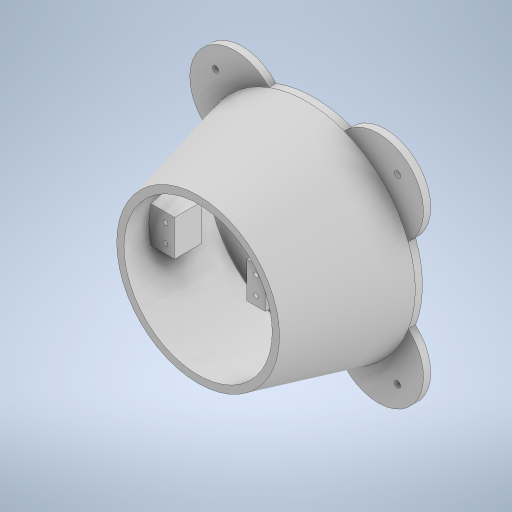
# Autodesk Inventor part: arm_base
Saved by Autodesk Inventor 2023 (Build 270158000, 158)
## iProperties
Created: 2023-01-17
Part Number: arm_base
Material: Generic
Document SubType Name: Modeling
Designer: denyh
Density: 1 g/cm^3
Appearance: Default
Author: denyh
Autodesk Inventor part; units mm, degrees
ref_plane "YZ Plane" through (0, 0, 0) normal (1, 0, 0) x (0, 1, 0)
ref_plane "XZ Plane" through (0, 0, 0) normal (0, 1, 0) x (-1, 0, 0)
ref_plane "Work Plane1" through (0, 0, 64) normal (0, 0, 1) x (1, 0, 0)
sketch "Sketch5" plane through (0, 0, 0) normal (0, 0, 1) x (1, 0, 0)
  circle A0 centre (0, 0) radius 60 projected
  line L0 (0, -6) -> (55.6072, -6) construction
  line L1 (0, 6) -> (55.6072, 6) construction
  arc A1 (-36.4842, -42.4842) -> (-36.4842, 42.4842) centre (0, 0) ccw
  circle A2 centre (0, 0) radius 56
  dimension "d15" = 6
  dimension "d16" = 12
  constraints: 4 end point, 2 horizontal, 2 point on circle, 1 centre point, 1 coincident, 3 other
  measures "d15" distance of A0.centre L1.start
  measures "d16" distance of L1.start L0.start
extrude "Extrusion1" add sketch "Sketch5" along normal blind 4 contours A0 | A2 A1
sketch "Sketch6" plane through (0, 0, 64) normal (0, 0, 1) x (1, 0, 0)
  circle A0 centre (0, 0) radius 45
  dimension "d22" = 90
  constraints: 1 centre point, 1 coincident
  measures "d22" diameter of A0
loft "Loft3" add profiles "Sketch6" section 1 edges at (-60, 0, 4)
sketch "Sketch9" plane through (0, 0, 64) normal (0, 0, 1) x (1, 0, 0)
  circle A0 centre (0, 0) radius 41
  dimension "d28" = 82
  constraints: 1 centre point, 1 coincident
  measures "d28" diameter of A0
sketch "Sketch10" plane through (0, 0, 0) normal (0, 0, -1) x (-1, 0, 0)
  circle A0 centre (0, 0) radius 56
  dimension "d29" = 112
  constraints: 1 centre point, 1 coincident
  measures "d29" diameter of A0
loft "Loft4" cut profiles "Sketch10", "Sketch9"
sketch "Sketch11" plane through (0, 0, 0) normal (0, 0, -1) x (-1, 0, 0)
  line L0 (0, 0) -> (0, 6)
  line L1 (0, 6) -> (-36.4842, 42.4842)
  circle A0 centre (0, 0) radius 56 projected
  line L2 (0, 0) -> (0, -6)
  line L3 (0, -6) -> (-36.4842, -42.4842)
  arc A1 (-36.4842, 42.4842) -> (-36.4842, -42.4842) centre (0, 0) ccw
  dimension "d34" = 6
  dimension "d35" = 135
  dimension "d36" = 6
  dimension "d37" = 135
  constraints: 8 end point, 4 point on circle, 2 vertical, 1 centre point, 1 coincident, 1 concentric
  measures "d34" distance of L0.start L0.end
  measures "d35" angle of L1 L0
  measures "d36" distance of L2.start L2.end
  measures "d37" angle of L2 L3
extrude "Extrusion2" add sketch "Sketch11" against normal blind 4 contours L2 L3 A0 L1 L0 picked at (-37.0571, 3.1994)
sketch "Sketch13" plane through (0, 0, 4) normal (0, 0, 1) x (1, 0, 0)
  line L0 (0, 0) -> (14, 0)
  line L1 (14, 0) -> (19, 0)
  line L2 (19, 0) -> (19, -10)
  line L3 (19, -10) -> (9, -10)
  line L4 (9, -10) -> (9, 10)
  line L5 (9, 10) -> (19, 10)
  line L6 (19, 10) -> (19, 0)
  dimension "d46" = 14
  dimension "d47" = 5
  dimension "d48" = 10
  dimension "d49" = 10
  dimension "d50" = 20
  constraints: 14 end point, 5 perpendicular, 2 point on line, 1 horizontal
  measures "d46" distance of L0.start L0.end
  measures "d47" distance of L0.end L1.end
  measures "d48" distance of L1.end L2.end
  measures "d49" distance of L2.end L3.end
  measures "d50" distance of L3.end L4.end
extrude "Extrusion3" add sketch "Sketch13" along normal blind 42
sketch "Sketch14" plane through (0, 0, 46) normal (0, 0, 1) x (1, 0, 0)
  line L0 (0, 0) -> (14, 0)
  line L1 (14, 0) -> (14, -5)
  circle A0 centre (14, -5) radius 1.3
  line L2 (14, 0) -> (14, 5)
  circle A1 centre (14, 5) radius 1.3
  dimension "d53" = 14
  dimension "d54" = 5
  dimension "d55" = 2.6
  dimension "d56" = 5
  dimension "d57" = 2.6
  constraints: 6 end point, 2 centre point, 2 coincident, 1 horizontal, 1 perpendicular, 1 vertical
  measures "d53" distance of L0.start L0.end
  measures "d54" distance of L0.end L1.end
  measures "d55" diameter of A0
  measures "d56" distance of L0.end L2.end
  measures "d57" diameter of A1
extrude "Extrusion4" cut sketch "Sketch14" against normal blind 10
sketch "Sketch15" plane through (0, 0, 4) normal (0, 0, 1) x (1, 0, 0)
  line L0 (14, 0) -> (-36, 0)
  line L1 (-36, 0) -> (-31, 0)
  line L2 (-31, 0) -> (-31, -10)
  line L3 (-36, 0) -> (-41, 0)
  line L4 (-31, -10) -> (-41, -10)
  line L5 (-41, -10) -> (-41, 10)
  line L6 (-41, 10) -> (-31, 10)
  line L7 (-31, 10) -> (-31, 0)
  point P0 (0, 0)
  dimension "d60" = 50
  dimension "d61" = 5
  dimension "d62" = 10
  dimension "d63" = 5
  dimension "d64" = 10
  dimension "d65" = 20
  constraints: 16 end point, 4 perpendicular, 3 horizontal, 1 point on line
  measures "d60" distance of L0.start L0.end
  measures "d61" distance of L0.end L1.end
  measures "d62" distance of L1.end L2.end
  measures "d63" distance of L0.end L3.end
  measures "d64" distance of L2.end L4.end
  measures "d65" distance of L4.end L5.end
extrude "Extrusion5" add sketch "Sketch15" along normal blind 42
chamfer "Chamfer1" distance 42 angle 5 1 edges at (14, 10, 4) measured on face at (14, 10, 4.5)
chamfer "Chamfer2" distance 42 angle 5 1 edges at (14, -10, 4) measured on face at (14, -10, 4.5)
sketch "Sketch18" plane through (9, -13.6745, 4) normal (-1, 0, 0) x (0, 0, 1)
  line L0 (42, 3.6745) -> (42, 23.6745) projected
  line L1 (32, 9.9745) -> (32, 7.3745) projected
  line L2 (0, 55.4938) -> (0, -28.1448) projected
  line L3 (10, 8.6745) -> (10, 18.6745)
  line L4 (32, 19.9745) -> (32, 17.3745) projected
  line L5 (10, 14.0291) -> (0, 14.0291)
  line L6 (10, 18.6745) -> (30, 18.6745)
  line L7 (30, 18.6745) -> (30, 8.6745)
  line L8 (30, 8.6745) -> (10, 8.6745)
  point P0 (-4, 13.6745)
  dimension "d87" = 10
  dimension "d88" = 10
  dimension "d89" = 20
  dimension "d90" = 10
  constraints: 10 end point, 3 perpendicular, 2 point on line, 1 horizontal
  measures "d87" distance of L3.start L3.end
  measures "d88" distance of L5.start L5.end
  measures "d89" distance of L3.end L6.end
  measures "d90" distance of L6.end L7.end
extrude "Extrusion8" cut sketch "Sketch18" along normal blind 16.6625 and the other way blind 11.9
ref_plane "Work Plane2" through (0, 0, 31) normal (0, 0, 1) x (1, 0, 0)
sketch "Sketch19" plane through (0, 0, 31) normal (0, 0, 1) x (1, 0, 0)
  line L0 (-31, -10) -> (-47.8184, -10)
  line L1 (-48.8154, -4.8836) -> (-48.7332, 5.4065)
  line L2 (-31, 10) -> (-41, 10) projected
  line L3 (-47.8184, 10) -> (-31, 10)
  line L4 (-31, 10) -> (-31, -10)
  line L5 (-48.7332, 5.4065) -> (-47.8184, 10)
  line L6 (-48.8154, -4.8836) -> (-47.8184, -10)
  point P0 (0, 0)
  constraints: 12 end point, 1 horizontal, 1 parallel, 1 perpendicular
extrude "Extrusion9" add sketch "Sketch19" along normal blind 15
sketch "Sketch20" plane through (-31, -10, 46) normal (1, 0, 0) x (0, 0, -1)
  line L0 (15, 0) -> (15, 20) projected
  line L1 (15, 0) -> (15, 20)
  line L2 (42, 20) -> (15, 20) projected
  line L3 (42, 20) -> (42, 0)
  line L4 (42, 70) -> (42, -50) projected
  line L5 (42, 0) -> (15, 0) projected
  line L6 (42, 0) -> (15, 0)
  point P0 (46, 10)
  constraints: 6 end point, 1 collinear, 1 point on line, 1 vertical
extrude "Extrusion10" cut sketch "Sketch20" against normal blind 12
fillet "Fillet1" radius 25 2 edges at (-48.4744, 5.0268, 31) (-48.4744, -5.0268, 31)
sketch "Sketch17" plane through (0, 0, 46) normal (0, 0, 1) x (1, 0, 0)
  line L0 (-31, -10) -> (-31, 10) projected
  line L1 (-31, 0) -> (-41, 0)
  line L2 (-41, 10) -> (-41, -10) projected
  line L3 (-36, 0) -> (-36, -5)
  line L4 (-36, -5) -> (-36, 5)
  circle A0 centre (-36, 5) radius 1.3
  circle A1 centre (-36, -5) radius 1.3
  point P0 (0, 0)
  dimension "d72" = 10
  dimension "d73" = 5
  dimension "d74" = 10
  dimension "d75" = 2.6
  dimension "d76" = 2.6
  constraints: 6 end point, 3 midpoint, 2 centre point, 2 coincident, 1 point on line, 1 vertical
  measures "d72" distance of L1.start L1.end
  measures "d73" distance of L3.start L3.end
  measures "d74" distance of L3.end L4.end
  measures "d75" diameter of A0
  measures "d76" diameter of A1
extrude "Extrusion7" cut sketch "Sketch17" against normal blind 10
sketch "Sketch21" plane through (0, 0, 4) normal (0, 0, 1) x (1, 0, 0)
  line L0 (19, 13.6745) -> (19, -13.6745) projected
  line L1 (19, -13.6745) -> (19, -8.1745)
  line L2 (19, -8.1745) -> (23, -8.1745)
  line L3 (23, -8.1745) -> (23, -9.1745)
  line L4 (23, -8.1745) -> (23, -7.1745)
  line L5 (23, -7.1745) -> (19, -7.1745)
  line L6 (23, -9.1745) -> (19, -9.1745)
  line L7 (19, 0) -> (24.9994, 0)
  line L8 (23, 8.1745) -> (23, 9.1745)
  line L9 (23, 8.1745) -> (23, 7.1745)
  line L10 (23, 7.1745) -> (19, 7.1745)
  line L11 (23, 9.1745) -> (19, 9.1745)
  point P0 (0, 0)
  dimension "d109" = 5.5
  dimension "d110" = 4
  dimension "d111" = 1
  dimension "d112" = 1
  constraints: 22 end point, 5 symmetric about line, 4 perpendicular, 3 point on line, 1 horizontal, 1 midpoint, 1 vertical
  measures "d109" distance of L0.end L1.end
  measures "d110" distance of L1.end L2.end
  measures "d111" distance of L2.end L3.end
  measures "d112" distance of L2.end L4.end
extrude "Extrusion11" add sketch "Sketch21" along normal blind 30
chamfer "Chamfer5" distance 30 angle 7 1 edges at (23, -8.1745, 34) measured on face at (23, -8.1745, 33.5)
chamfer "Chamfer6" distance 30 angle 7 1 edges at (23, 8.1745, 34) measured on face at (23, 8.1745, 33.5)
sketch "Sketch23" plane through (0, 0, 0) normal (0, 0, -1) x (-1, 0, 0)
  line L0 (0, 0) -> (58.0755, -58.0755)
  line L1 (0, 0) -> (82.1312, 0) construction
  arc A0 (-36.4842, -42.4842) -> (-36.4842, 42.4842) centre (0, 0) ccw projected
  circle A1 centre (39.598, -39.598) radius 25
  circle A2 centre (50.2576, -50.2576) radius 1.7
  circle A3 centre (39.598, 39.598) radius 25
  circle A4 centre (50.2576, 50.2576) radius 1.7
  circle A5 centre (-39.598, 39.598) radius 25
  circle A6 centre (-50.2576, 50.2576) radius 1.7
  circle A7 centre (-39.598, -39.598) radius 25
  circle A8 centre (-50.2576, -50.2576) radius 1.7
  circle A9 centre (0, 0) radius 45
  circle A10 centre (0, 0) radius 36
  point P0 (42.5078, -14.7679)
  point P1 (42.5078, 14.7679)
  point P2 (14.7679, 42.5078)
  point P3 (-14.7679, 42.5078)
  point P4 (-42.5078, 14.7679)
  point P5 (-42.5078, -14.7679)
  point P6 (-14.7679, -42.5078)
  point P7 (14.7679, -42.5078)
  dimension "d122" = 45
  dimension "d123" = 50
  dimension "d124" = 3.4
  dimension "d127" = 360
  dimension "d129" = 90
  dimension "d130" = 72
  constraints: 10 centre point, 4 end point, 2 coincident, 2 point on line, 1 equal length, 1 horizontal, 1 point on circle, 17 other
  measures "d122" angle of L0 L1
  measures "d123" diameter of A1
  measures "d124" diameter of A2
  measures "d129" diameter of A9
  measures "d130" diameter of A10
extrude "Extrusion12" add sketch "Sketch23" against normal blind 4 contours A10 A1 A9 L0 | L0 A9 A1 A10 | A10 A3 A9 A1 | A1 A9 A7 A10 | A9 A1 A0 L0 | L0 A0 A1 A9 | A7 A9 A10 | A0 A1 L0 A2 | L0 A2 A1 A0 | A10 A3 A9 | A7 A9 | A7 A9 A5 A10 | A3 A9 A0 | A0 A3 | A10 A5 A9 A3 | A5 A9 A10 | A5 A9
body "Solid2"
